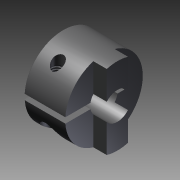
# Autodesk Inventor part: MCOC17-6_c
Saved by Autodesk Inventor 2015 SP1 (Build 190203100, 203)
## iProperties
Category: PARTsolutions
Company: MISUMI
Created: 2015-02-02
Part Number: MCOC17-6_c
Catalog Web Link: http://us.misumi-ec.com/vona2/detail/110300123930
Description: MCOC_coup-Couplings - Oldham Clamping Type
Vendor: MISUMI
Document SubType Name: Modeling
Designer: PARTuser1
Manufacturer: MISUMI
Mass: 1.68591 g
Surface Area: 13.3267 cm^2
Volume: 1.68591 cm^3
Density: 1 g/cm^3
Material: Generic
Appearance: PSOLRGB-192-192-192
Stock Number: MCOC17-5-6
PSOL_IDENT_0: {\\10.0.0.236\data_v8\23d-libs\misumi\metric\50_couplings\parts\mcoc_coup.prj},198 {VTYP=3D},{NB=MCO
PSOL_IDENT_1: C17-6_c},{LINA=MCOC17-6},{NN=MCOC_coup},{DATE=13.11.2014 06:59:38},{GEOMDATE=05.12.2013 00:00:00},{V
PSOL_IDENT_2: ERSION=},{LINEID=1040},{LINESUBID=-1},{WBVAR=HS,KGHS,ALT1,LDC,ALT2,RDC,DD,KGWC}  {NB=MCOC17-6_c},{LI
PSOL_IDENT_3: NA=MCOC17-6},{KT=DUMMY},{PN=MCOC17-6},{HS=MCOC},{KGHS=},{KGHSALG='','N/A'},{MATH=304 Stainless Steel
PSOL_IDENT_4: Sintered Alloy},{MATS=Carbon Reinforced Resin},{AC=Hexagon Socket Head Cap Screw},{TYPE=MCOC},{NO=1
PSOL_IDENT_5: 7},{ALT1=},{ALT1ALG=},{ALT13D=6},{DLALT1=6},{LDC=0.00},{LDCMIN=5},{LDCALG=0},{ALT2=},{ALT2ALG=},{ALT
PSOL_IDENT_6: 2ALG1= '', 'w/o RDC (Shaft Hole Diameter Right Shaft)','RDC','with RDC (Shaft Hole Diameter Right Sh
PSOL_IDENT_7: aft)'},{ALT23D=6},{RDC=0.00},{RDCALG=[0]},{DD=6.00},{DDALG=5,6,6.35},{DDPN=-6},{D=16.8},{D1=17.5},{D
PSOL_IDENT_8: 2=19},{DD3=7.2},{L=24.4},{LL=9.0},{A=5.0},{F=4.0},{M=M3},{T=1.8},{ALTALG2='','Select RDC'},{HSALG='M
PSOL_IDENT_9: COC','Standard Hole','','Key Groove Hole'},{TSIMD=3},{R1=5.5},{SC1=3.000},{SC2=5.000},{B=3.500},{L9=
PSOL_IDENT_10: 0.800},{W=4.600},{G=2.900},{TT=1},{BB=2},{HSX=MCOC},{Z=4.440},{Z1=1.200},{KGWC=},{KGWCALG= '' , 'N/A'
PSOL_IDENT_11: },{KGWCPN=},{KGWC1=0},{TTKGW=0.0},{CIF=0},{BL=10}
SUPPLIER: MISUMI
ARTICLENO: MCOC17-6_c
BOMINFO: MCOC17-6
CREATOR: CADENAS GmbH
Title: MCOC17-6
Author: Misumi
Comments: Couplings - Oldham Clamping Type
Autodesk Inventor part; units mm, degrees
sketch "Sketch_1" plane through (0, 0, 0) normal (0, 0, 1) x (1, 0, 0)
  line L0 (11.9, 0) -> (0, 0)
  line L1 (0, 0) -> (0, 8.2)
  line L2 (0, 8.2) -> (0.2, 8.4)
  line L3 (0.2, 8.4) -> (11.9, 8.4)
  line L4 (11.9, 8.4) -> (11.9, 0)
  line L5 (11.9, 0) -> (0, 0)
  constraints: 12 end point
revolve "Revolution1" add sketch "Sketch_1" angle 360 about axis through (11.9, 0, 0) along (1, 0, 0)
sketch "Sketch_6" plane through (0, 0, 0) normal (1, 0, 0) x (0, 1, 0)
  line L0 (0, 0.6) -> (-8.4, 0.6)
  line L1 (-8.4, 0.6) -> (-8.4, -0.6)
  line L2 (-8.4, -0.6) -> (0, -0.6)
  line L3 (0, -0.6) -> (0, 0.6)
  constraints: 8 end point
extrude "Extrusion1" cut sketch "Sketch_6" along normal blind 9
sketch "Sketch_7" plane through (4, 0, 0) normal (1, 0, 0) x (0, 0, -1)
  line L0 (-8.4, -5) -> (8.4, -5)
  line L1 (8.4, -5) -> (8.4, -7.75)
  line L2 (8.4, -7.75) -> (3, -7.75)
  line L3 (3, -7.75) -> (3, -6.5)
  line L4 (3, -6.5) -> (0.6, -6.5)
  line L5 (0.6, -6.5) -> (0.6, -5)
  line L6 (0.6, -5) -> (8.4, -5)
  constraints: 14 end point
revolve "Revolution2" cut sketch "Sketch_7" angle 360 about axis through (4, -5, 8.4) along (0, 0, 1)
sketch "Sketch_13" plane through (4, 0, 0) normal (1, 0, 0) x (0, 0, -1)
  line L0 (-8.4, -5) -> (8.4, -5)
  line L1 (-0.6, -5) -> (-0.6, -6.2295)
  line L2 (-0.6, -6.2295) -> (-8.4, -6.2295)
  line L3 (-8.4, -6.2295) -> (-8.4, -5)
  line L4 (-8.4, -5) -> (-0.6, -5)
  constraints: 10 end point
revolve "Revolution3" cut sketch "Sketch_13" angle 360 about axis through (4, -5, 8.4) along (0, 0, 1)
thread "Thread1" size "M3x0.5" class "6H" standard "ISO Metric profile" length 4.7207 offset 2.1855
sketch "Sketch_2" plane through (11.9, 0, 0) normal (1, 0, 0) x (0, 0, -1)
  line L0 (-9.4, 8.9) -> (-9.4, -8.9)
  line L1 (-9.4, -8.9) -> (9.4, -8.9)
  line L2 (9.4, -8.9) -> (9.4, 8.9)
  line L3 (9.4, 8.9) -> (-9.4, 8.9)
  line L4 (-8.4, 2.3) -> (-8.4, -2.3)
  line L5 (-8.4, -2.3) -> (8.4, -2.3)
  line L6 (8.4, -2.3) -> (8.4, 2.3)
  line L7 (8.4, 2.3) -> (-8.4, 2.3)
  constraints: 16 end point
extrude "Extrusion2" cut sketch "Sketch_2" against normal blind 2.9
sketch "Sketch_3" plane through (0, 0, 0) normal (0, 0, 1) x (1, 0, 0)
  line L0 (11.9, 0) -> (0, 0)
  line L1 (0, 0) -> (0, 3)
  line L2 (0, 3) -> (11.9, 3)
  line L3 (11.9, 3) -> (11.9, 0)
  line L4 (11.9, 0) -> (0, 0)
  constraints: 10 end point
revolve "Revolution4" cut sketch "Sketch_3" angle 360 about axis through (11.9, 0, 0) along (1, 0, 0)
sketch "Sketch_17" plane through (0, 0, 0) normal (1, 0, 0) x (0, 0, -1)
  line L0 (-0.6, 0) -> (0.6, 0)
  line L1 (0.6, 0) -> (0.6, 4.44)
  line L2 (0.6, 4.44) -> (-0.6, 4.44)
  line L3 (-0.6, 4.44) -> (-0.6, 0)
  constraints: 8 end point
extrude "Extrusion3" cut sketch "Sketch_17" along normal blind 11.9
ref_plane "L_XY" through (12.2, 0, 0) normal (1, 0, 0) x (0, 0, -1)
ref_plane "L_YZ" through (12.2, 0, 0) normal (0, 0, -1) x (0, 1, 0)
ref_plane "L_ZX" through (12.2, 0, 0) normal (0, 1, 0) x (1, 0, 0)
ref_plane "screw_XY" through (4, -5, -3) normal (0, 0, -1) x (1, 0, 0)
ref_plane "screw_YZ" through (4, -5, -3) normal (1, 0, 0) x (0, -1, 0)
ref_plane "screw_ZX" through (4, -5, -3) normal (0, -1, 0) x (0, 0, -1)
body "Solid1"
